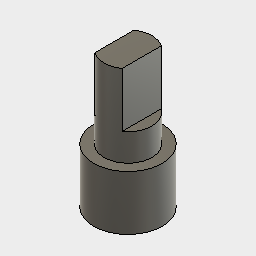
Encoder Shaft (Autodesk Fusion 360 design; units mm, degrees)
Autodesk Fusion 360 part; units mm, degrees
sketch "Base Sketch" plane through (0, 0, 0) normal (0, 1, 0) x (1, 0, 0)
  circle A0 centre (0, 0) radius 2.5 construction
  line L0 (-1.8028, 3) -> (1.8028, 3) construction
  line L1 (-1.8028, -3) -> (1.8028, -3) construction
  arc A1 (-1.8028, 3) -> (-1.8028, -3) centre (0, 0) ccw construction
  arc A2 (1.8028, -3) -> (1.8028, 3) centre (0, 0) ccw construction
  line L2 (-5, 5) -> (8, 5) construction
  line L3 (8, 5) -> (8, -5) construction
  line L4 (8, -5) -> (-5, -5) construction
  line L5 (-5, -5) -> (-5, 5) construction
  line L6 (8, 6) -> (-6, 6) construction
  line L7 (-6, 6) -> (-6, -6) construction
  line L8 (-6, -6) -> (8, -6) construction
  line L9 (8, -6) -> (8, 6) construction
  line L10 (8, 2.5) -> (6, 2.5) construction
  line L11 (6, 2.5) -> (6, 1.5) construction
  line L12 (6, 1.5) -> (8, 1.5) construction
  line L13 (8, 1.5) -> (8, 2.5) construction
  line L14 (8, -1.5) -> (6, -1.5) construction
  line L15 (6, -1.5) -> (6, -2.5) construction
  line L16 (6, -2.5) -> (8, -2.5) construction
  line L17 (8, -2.5) -> (8, -1.5) construction
  line L18 (-5, -6) -> (-1, -6) construction
  line L19 (-1, -6) -> (-1, -4) construction
  line L20 (-1, -4) -> (-5, -4) construction
  line L21 (-5, -4) -> (-5, -6) construction
  line L22 (2.5, 6) -> (6.5, 6) construction
  line L23 (6.5, 6) -> (6.5, 4) construction
  line L24 (6.5, 4) -> (2.5, 4) construction
  line L25 (2.5, 4) -> (2.5, 6) construction
  circle A3 centre (-20.5, 0) radius 8.5 construction
  circle A4 centre (-20.5, 0) radius 10 construction
  line L26 (8, 8) -> (-29, 8) construction
  line L27 (-29, 8) -> (-29, -8) construction
  line L28 (-29, -8) -> (8, -8) construction
  line L29 (8, -8) -> (8, 8) construction
  dimension "d1" = 5
  dimension "d2" = 7
  dimension "d3" = 6
  dimension "d4" = 3
  dimension "d5" = 10
  dimension "d6" = 5
  dimension "d7" = 5
  dimension "d8" = 13
  dimension "d9" = 1
  dimension "d10" = 1
  dimension "d11" = 1
  dimension "d12" = 2.5
  dimension "d13" = 2.5
  dimension "d14" = 1
  dimension "d15" = 2
  dimension "d16" = 4
  dimension "d17" = 2
  dimension "d18" = 4
  dimension "d19" = 2
  dimension "d20" = 7.5
  dimension "d21" = 17
  dimension "d22" = 1.5
  dimension "d23" = 4.5
  dimension "d24" = 37
  dimension "d25" = 16
  constraint coincident A0.centre A1.centre
  constraint horizontal L0
  constraint coincident A0.centre A1
  constraint parallel L0 L1
  constraint concentric A1 A2
  constraint horizontal L2
  constraint vertical L3
  constraint horizontal L4
  constraint vertical L5
  constraint horizontal L6
  constraint vertical L7
  constraint horizontal L8
  constraint vertical L9
  constraint collinear L3 L9
  constraint horizontal L10
  constraint vertical L11
  constraint horizontal L12
  constraint vertical L13
  constraint coincident L3 A0.centre
  constraint horizontal L14
  constraint vertical L15
  constraint horizontal L16
  constraint vertical L17
  constraint equal L10 L14
  constraint equal L11 L15
  constraint horizontal L18
  constraint vertical L19
  constraint horizontal L20
  constraint vertical L21
  constraint coincident L8 A0.centre
  constraint collinear L5 L21
  constraint horizontal L22
  constraint vertical L23
  constraint horizontal L24
  constraint vertical L25
  constraint coincident L6 A0.centre
  constraint horizontal A0.centre A1.centre
  constraint concentric A3 A4
  constraint coincident A4 A0.centre
  constraint horizontal L26
  constraint vertical L27
  constraint horizontal L28
  constraint vertical L29
  constraint collinear L3 L29
  constraint coincident L27 A0.centre
  constraint midpoint L27 A0.centre
  measures "d1" diameter of A0
  measures "d2" diameter of A1
  measures "d3" distance of L0 L1
  measures "d9" distance of L2 L6
  measures "d10" distance of L5 L7
  measures "d11" distance of L4 L8
  measures "d12" distance of L2 L10
  measures "d13" distance of L4 L16
  measures "d14" distance of A0.centre
  measures "d20" distance of L5 L25
  measures "d21" diameter of A3
  measures "d22" distance of A3 A4
sketch "Sketch10" plane through (0, 0, 0) normal (0, 1, 0) x (1, 0, 0)
  line L0 (-3.25, 2.6) -> (3.25, 2.6) construction
  line L1 (3.25, 2.6) -> (3.25, -2.6) construction
  line L2 (3.25, -2.6) -> (-3.25, -2.6) construction
  line L3 (-3.25, -2.6) -> (-3.25, 2.6) construction
  line L4 (-3.25, 2.6) -> (3.25, -2.6) construction
  line L5 (-5, 5) -> (6, 5) construction
  line L6 (6, 5) -> (6, -5) construction
  line L7 (6, -5) -> (-5, -5) construction
  line L8 (-5, -5) -> (-5, 5) construction
  line L9 (8, -5) -> (-5, -5) construction
  line L10 (6, -1.5) -> (6, -2.5) construction
  line L11 (6, 1.5) -> (8, 1.5) construction
  line L12 (8, 1.5) -> (8, -1.5) construction
  line L13 (8, -1.5) -> (6, -1.5) construction
  line L14 (6, -1.5) -> (6, 1.5) construction
  circle A0 centre (0, 0) radius 2.5 construction
  circle A1 centre (0, 0) radius 2.5 construction
  circle A2 centre (0, 0) radius 2.5 construction
  dimension "d56" = 6.5
  dimension "d57" = 5.2
  constraint horizontal L0
  constraint vertical L1
  constraint horizontal L2
  constraint vertical L3
  constraint midpoint L4 A0.centre
  constraint horizontal L5
  constraint vertical L6
  constraint horizontal L7
  constraint vertical L8
  constraint coincident A0.centre L9
  constraint coincident A0.centre A1.centre
  constraint collinear L6 L10
  constraint horizontal L11
  constraint vertical L12
  constraint horizontal L13
  constraint vertical L14
  constraint equal A0 A2
sketch "Sketch11" plane through (0, 0, 0) normal (0, 1, 0) x (1, 0, 0)
  circle A0 centre (5, 4) radius 1 construction
  circle A1 centre (-4, -4) radius 1 construction
  line L0 (-5, 5) -> (6, 5)
  line L1 (-3.25, 2.6) -> (3.25, 2.6) construction
  line L2 (3.25, -2.6) -> (-3.25, -2.6) construction
  line L3 (6, -5) -> (-5, -5)
  circle A2 centre (5, 4) radius 0.5 construction
  circle A3 centre (-4, -4) radius 0.5 construction
  line L4 (-4, 4) -> (5, 4) construction
  line L5 (5, 4) -> (5, -4) construction
  line L6 (5, -4) -> (-4, -4) construction
  line L7 (-4, -4) -> (-4, 4) construction
  line L8 (-5, -5) -> (-5, 5)
  line L9 (6, -1.5) -> (6, 1.5) construction
  dimension "d58" = 2
  dimension "d59" = 2
  dimension "d60" = 1
  dimension "d61" = 1
  dimension "d62" = 1
  dimension "d63" = 1
  dimension "d64" = 1
  dimension "d65" = 1
  constraint concentric A0 A2
  constraint concentric A1 A3
  constraint horizontal L4
  constraint vertical L5
  constraint horizontal L6
  constraint vertical L7
  measures "d58" diameter of A0
  measures "d59" diameter of A1
  measures "d60" diameter of A2
  measures "d61" diameter of A3
  measures "d62" distance of L0 L4
  measures "d63" distance of L3 L6
  measures "d64" distance of L7 L8
  measures "d65" distance of L5 L9
sketch "Sketch12" plane through (0, 0, 0) normal (0, 1, 0) x (1, 0, 0)
  circle A0 centre (5, 4) radius 1
  circle A1 centre (5, 4) radius 1
  circle A2 centre (-4, -4) radius 1
  circle A3 centre (-4, -4) radius 1
sketch "Sketch17" plane through (0, 0, 0) normal (0, 1, 0) x (1, 0, 0)
  circle A0 centre (0, 0) radius 2.5
  dimension "d77" = 5
  constraint coincident A0.centre origin
  measures "d77" diameter of A0
extrude "Extrude14" add sketch "Sketch17" along normal blind 4
sketch "Sketch18" plane through (0, 4, 0) normal (0, 1, 0) x (-1, 0, 0)
  circle A0 centre (0, 0) radius 2.5
  circle A1 centre (0, 0) radius 1.75
  dimension "d80" = 3.5
  constraint coincident A0.centre A1.centre
  measures "d80" diameter of A1
extrude "Extrude15" add sketch "Sketch18" along normal blind 2 contours A1
sketch "Sketch19" plane through (0, 6, 0) normal (0, 1, 0) x (-1, 0, 0)
  circle A0 centre (0, 0) radius 1.75
  line L0 (1, 0) -> (-1, 0)
  line L1 (1, -1.4361) -> (1, 1.4361)
  line L2 (-1, -1.4361) -> (-1, 1.4361)
  arc A1 (-1, -1.4361) -> (1, -1.4361) centre (0, 0) ccw
  arc A2 (1, 1.4361) -> (-1, 1.4361) centre (0, 0) ccw
  dimension "d83" = 2
  constraint coincident A0.centre A1.centre
  constraint equal A0 A1
  constraint horizontal L0
  constraint midpoint A0.centre L0
  constraint coincident A0.centre A1
  constraint midpoint A0.centre L2
  constraint midpoint A0.centre L1
  constraint concentric A1 A2
extrude "Extrude16" add sketch "Sketch19" along normal blind 4 contours A0 L0 L1 L2 A2 | A0 L0 L1 L2 A1
